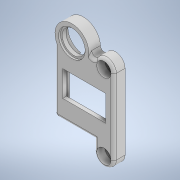
# Autodesk Inventor part: Oberschale
Saved by Autodesk Inventor 2020.2 (Build 242310000, 310)
## iProperties
Created: 2020-05-20
Part Number: Oberschale
Material: Generisch
Document SubType Name: Modeling
Designer: hpcwoess
Density: 1 g/cm^3
Appearance: Vorgabe
Author: hpcwoess
Autodesk Inventor part; units mm, degrees
ref_plane "YZ Plane" through (0, 0, 0) normal (1, 0, 0) x (0, 1, 0)
ref_plane "XZ Plane" through (0, 0, 0) normal (0, 1, 0) x (-1, 0, 0)
ref_plane "XY Plane" through (0, 0, 0) normal (0, 0, 1) x (1, 0, 0)
sketch "Skizze1" plane through (0, 0, 0) normal (0, 0, 1) x (1, 0, 0)
  line L0 (-15.2, 13.5) -> (-1.0671, 13.5)
  line L1 (15.2, 17) -> (15.2, -15.8)
  line L2 (-15.2, -16.5) -> (-15.2, 13.5)
  line L3 (-11.2, 6.7) -> (11.2, 6.7)
  line L4 (11.2, 6.7) -> (11.2, -6.7)
  line L5 (11.2, -6.7) -> (-11.2, -6.7)
  line L6 (-11.2, -6.7) -> (-11.2, 6.7)
  circle A0 centre (-6.4, 20.5) radius 6
  arc A1 (2.3937, 20.8323) -> (-15.2, 20.5) centre (-6.4, 20.5) ccw
  line L7 (-15.2, 13.5) -> (-15.2, 20.5)
  arc A2 (15.2, 17) -> (6.0516, 19.7913) centre (10.2, 17) ccw
  arc A3 (2.3937, 20.8323) -> (6.0516, 19.7913) centre (4.3923, 20.9078) ccw
  circle A4 centre (10.2, 17) radius 2.3
  circle A5 centre (10.2, -22) radius 2.3
  arc A6 (5.2, -22) -> (15.2, -22) centre (10.2, -22) ccw
  line L8 (15.2, -15.8) -> (15.2, -22)
  line L9 (5.2, -22) -> (5.2, -16.5)
  line L10 (5.2, -16.5) -> (-15.2, -16.5)
  point P0 (0, 0)
  dimension "d0" = 22.4
  dimension "d1" = 11.2
  dimension "d3" = 15.2
  dimension "d4" = 13.4
  dimension "d5" = 6.7
  dimension "d8" = 6.8
  dimension "d32" = 12
  dimension "d33" = 17.6
  dimension "d34" = 7
  dimension "d35" = 8.8
  dimension "d36" = 10
  dimension "d37" = 3.5
  dimension "d38" = 4
  dimension "d39" = 4.6
  dimension "d40" = 4.6
  dimension "d41" = 10
  dimension "d43" = 30
  dimension "d61" = 9.8
  dimension "d62" = 15.2
  dimension "d65" = 5
  dimension "d66" = 39
  dimension "d67" = 17
  constraints: 22 end point, 8 point on circle, 7 centre point, 6 tangent, 4 parallel, 3 coincident, 3 perpendicular, 2 horizontal
  measures "d0" distance between parallel lines of L4 L6
  measures "d1" distance from line of L4 point (0, 0)
  measures "d3" distance from line of L2 point (0, 0)
  measures "d4" distance between parallel lines of L5 L3
  measures "d5" distance from line of L5 point (0, 0)
  measures "d8" distance between parallel lines of L0 L3
  measures "d32" diameter of A0
  measures "d33" diameter of A1
  measures "d34" distance from line of L0 A0.centre
  measures "d35" distance from line of A0.centre L2
  measures "d36" diameter of A2
  measures "d37" distance from line of L0 A2.centre
  measures "d38" diameter of A3
  measures "d39" diameter of A4
  measures "d40" diameter of A5
  measures "d41" diameter of A6
  measures "d43" distance between parallel lines of L10 L0
  measures "d61" distance between parallel lines of L5 L10
  measures "d62" distance from line of L1 point (0, 0)
  measures "d65" distance from line of A2.centre L1
  measures "d66" distance of A5.centre A2.centre
  measures "d67" vertical distance of A2.centre point (0, 0)
extrude "Extrusion1" add sketch "Skizze1" along normal blind 6
sketch "Skizze2" plane through (0, 0, 0) normal (0, 0, -1) x (-1, 0, 0)
  line L0 (-12.7, 7.5) -> (12.7, 7.5)
  line L1 (12.7, 7.5) -> (12.7, -10.1)
  line L2 (12.7, -10.1) -> (-12.7, -10.1)
  line L3 (-12.7, -10.1) -> (-12.7, 7.5)
  line L4 (11.2, 6.7) -> (-11.2, 6.7) projected
  line L5 (-4.5, -10.1) -> (4.5, -10.1)
  line L6 (4.5, -10.1) -> (4.5, -15)
  line L7 (4.5, -15) -> (-4.5, -15)
  line L8 (-4.5, -15) -> (-4.5, -10.1)
  line L9 (-6, 12.3) -> (6, 12.3)
  line L10 (6, 12.3) -> (6, 9.5)
  line L11 (6, 9.5) -> (-6, 9.5)
  line L12 (-6, 9.5) -> (-6, 12.3)
  line L13 (15.2, -16.5) -> (-5.2, -16.5) projected
  point P0 (0, 0)
  point P1 (4.5, -10.1)
  dimension "d11" = 25.4
  dimension "d12" = 17.6
  dimension "d24" = 9
  dimension "d25" = 4.5
  dimension "d26" = 12
  dimension "d27" = 6
  dimension "d28" = 2.8
  dimension "d29" = 2
  dimension "d44" = 6.4
  dimension "d45" = 12.7
  dimension "d46" = 4.9
  constraints: 24 end point, 6 parallel, 3 horizontal, 3 perpendicular, 1 point on line
  measures "d11" distance of L0.start L0.end
  measures "d12" distance of L0.end L1.end
  measures "d24" distance between parallel lines of L8 L6
  measures "d25" distance from line of L6 point (0, 0)
  measures "d26" distance between parallel lines of L10 L12
  measures "d27" distance from line of L10 point (0, 0)
  measures "d28" distance between parallel lines of L9 L11
  measures "d29" distance between parallel lines of L0 L11
  measures "d44" distance between parallel lines of L2 L13
  measures "d45" distance from line of L1 point (0, 0)
  measures "d46" distance between parallel lines of L5 L7
extrude "Extrusion2" cut sketch "Skizze2" against normal blind 4
sketch "Skizze3" plane through (0, 0, 0) normal (0, 0, -1) x (-1, 0, 0)
  line L0 (-13.7, 12.5) -> (13.7, 12.5)
  line L1 (13.7, 12.5) -> (13.7, -15.3)
  line L2 (13.7, -15.3) -> (-13.7, -15.3)
  line L3 (-13.7, -15.3) -> (-13.7, 12.5)
  line L4 (15.2, 20.5) -> (15.2, -16.5) projected
  line L5 (-15.2, -22) -> (-15.2, 17) projected
  line L6 (15.2, -16.5) -> (-5.2, -16.5) projected
  point P0 (0, 0)
  point P1 (-14.5619, 17.7435)
  dimension "d19" = 1.5
  dimension "d20" = 1.5
  dimension "d54" = 1.2
  dimension "d55" = 27.8
  constraints: 8 end point, 2 parallel, 1 horizontal, 1 perpendicular, 1 other
  measures "d19" distance between parallel lines of L4 L1
  measures "d54" distance between parallel lines of L6 L2
  measures "d55" distance between parallel lines of L2 L0
extrude "Extrusion3" cut sketch "Skizze3" against normal blind 2.2
fillet "Rundung1" radius 1.5 2 edges at (15.2, 17, 3) (-15.2, -16.5, 3)
fillet "Rundung2" radius 1.5 3 edges at (-14.7607, -16.0607, 6) (-15.2, 2.75, 6) (15.2, -2.5, 6)
sketch "Skizze4" plane through (0, 0, 6) normal (0, 0, 1) x (1, 0, 0)
  circle A0 centre (10.2, 17) radius 2.3 projected
  circle A1 centre (10.2, 17) radius 3.7
  circle A2 centre (10.2, -22) radius 2.3 projected
  circle A3 centre (10.2, -22) radius 3.7
  point P0 (0, 0)
  dimension "d47" = 7.4
  dimension "d48" = 7.4
  constraints: 2 centre point, 2 coincident
  measures "d47" diameter of A1
  measures "d48" diameter of A3
extrude "Extrusion4" cut sketch "Skizze4" against normal blind 4.2 contours A0 | A1 | A2 | A3
sketch "Skizze5" plane through (0, 0, 0) normal (0, 0, -1) x (-1, 0, 0)
  circle A0 centre (6.4, 20.5) radius 6 projected
  circle A1 centre (6.4, 20.5) radius 8.1
  point P0 (0, 0)
  dimension "d51" = 16.2
  constraints: 1 centre point, 1 coincident
  measures "d51" diameter of A1
extrude "Extrusion5" cut sketch "Skizze5" against normal blind 3
sketch "Skizze6" plane through (0, 0, 6) normal (0, 0, 1) x (1, 0, 0)
  circle A0 centre (-6.4, 20.5) radius 6 projected
  circle A1 centre (-6.4, 20.5) radius 8.8
  point P0 (0, 0)
  constraints: 1 centre point, 1 coincident
extrude "Extrusion6" add sketch "Skizze6" against normal blind 2
sketch "Skizze7" plane through (0, 0, 6) normal (0, 0, 1) x (1, 0, 0)
  circle A0 centre (-6.4, 20.5) radius 6 projected
  circle A1 centre (-6.4, 20.5) radius 6.9
  point P0 (0, 0)
  dimension "d58" = 13.8
  constraints: 1 centre point, 1 coincident
  measures "d58" diameter of A1
extrude "Extrusion7" cut sketch "Skizze7" against normal blind 1 contours A0 | A1
equation "\"d1\" = 0.5 * d0"
equation "\"d3\" = 0.5 * d2"
equation "\"d5\" = 0.5 * d4"
equation "\"d35\" = 0.5 * d33"
equation "\"d40\" = d39"
equation "\"d41\" = d36"
equation "\"d25\" = 0.5 * d24"
equation "\"d27\" = 0.5 * d26"
equation "\"d45\" = 0.5 * d11"
equation "\"d48\" = d47"
equation "\"d42\" = d37"
equation "\"d2\" = 30.4"
